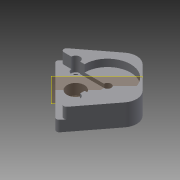
# Autodesk Inventor part: leveling clip
Saved by Autodesk Inventor 2014 (Build 180170000, 170)
## iProperties
Created: 2016-05-11
Part Number: leveling clip
Material: Generic
Document SubType Name: Modeling
Designer: eric.parent
Density: 1 g/cm^3
Appearance: Default
Author: eric.parent
Autodesk Inventor part; units mm, degrees
ref_plane "YZ Plane" through (0, 0, 0) normal (1, 0, 0) x (0, 1, 0)
ref_plane "XZ Plane" through (0, 0, 0) normal (0, 1, 0) x (-1, 0, 0)
ref_plane "XY Plane" through (0, 0, 0) normal (0, 0, 1) x (1, 0, 0)
sketch "Sketch1" plane through (0, 0, 0) normal (0, 0, 1) x (1, 0, 0)
  line L0 (202, 202) -> (202, 0) construction
  line L1 (0, 202) -> (202, 202) construction
  arc A0 (206.2012, 222.0831) -> (193.0425, 222.9456) centre (199.1301, 215.012) ccw projected
  arc A1 (222.9456, 193.0425) -> (222.0831, 206.2012) centre (215.012, 199.1301) ccw projected
  line L2 (206.2012, 222.0831) -> (222.0831, 206.2012)
  line L3 (193.0425, 222.9456) -> (165.7457, 202)
  line L4 (202, 165.7457) -> (222.9456, 193.0425)
  line L5 (165.7457, 202) -> (202, 165.7457)
  point P0 (0, 0)
  constraints: 8 end point, 3 tangent, 2 point on line, 1 parallel
extrude "Extrusion3" add sketch "Sketch1" along normal blind 15
sketch "Sketch3" plane through (0, 0, 15) normal (0, 0, 1) x (1, 0, 0)
  line L0 (165.7457, 202) -> (202, 202)
  line L1 (202, 202) -> (202, 165.7457)
  line L2 (165.7457, 202) -> (202, 165.7457)
  point P0 (0, 0)
  constraints: 6 end point, 1 horizontal, 1 perpendicular
extrude "Extrusion4" cut sketch "Sketch3" against normal blind 7.5
sketch "Sketch5" plane through (0, 0, 15) normal (0, 0, 1) x (1, 0, 0)
  line L0 (222.0831, 206.2012) -> (206.2012, 222.0831) construction
  line L1 (214.1421, 214.1421) -> (134.2284, 134.2284) construction
  line L2 (202, 165.7457) -> (165.7457, 202) construction
  circle A0 centre (190.9439, 190.9439) radius 6
  point P0 (0, 0)
  dimension "d25" = 12
  dimension "d26" = 10
  constraints: 2 end point, 1 centre point, 1 midpoint, 1 perpendicular, 1 point on line
  measures "d25" diameter of A0
  measures "d26" distance from line of L2 A0.centre
extrude "Extrusion6" cut sketch "Sketch5" against normal through all
sketch "Sketch6" plane through (0, 0, 15) normal (0, 0, 1) x (1, 0, 0)
  circle A0 centre (202, 202) radius 2.5
  point P0 (0, 0)
  dimension "d27" = 5
  constraints: 1 centre point, 1 coincident
  measures "d27" diameter of A0
extrude "Extrusion7" cut sketch "Sketch6" against normal through all
sketch "Sketch7" plane through (0, 0, 15) normal (0, 0, 1) x (1, 0, 0)
  arc A0 (202, 199.5) -> (199.5, 202) centre (202, 202) ccw construction
  circle A1 centre (202, 202) radius 16
  point P0 (0, 0)
  dimension "d30" = 32
  constraints: 1 centre point, 1 coincident
  measures "d30" diameter of A1
extrude "Extrusion8" cut sketch "Sketch7" against normal blind 5
sketch "Sketch8" plane through (0, 0, 15) normal (0, 0, 1) x (1, 0, 0)
  line L0 (202, 186) -> (202, 165.7457) construction
  circle A0 centre (190.9439, 190.9439) radius 6 construction
  line L1 (202, 165.7457) -> (165.7457, 202) construction
  line L2 (163.0953, 218.7925) -> (219.2426, 162.6452) construction
  circle A1 centre (202, 179.8878) radius 1.65
  point P0 (0, 0)
  dimension "d33" = 3.3
  constraints: 3 point on line, 2 end point, 1 centre point, 1 parallel
  measures "d33" diameter of A1
extrude "Extrusion9" cut sketch "Sketch8" against normal through all
sketch "Sketch9" plane through (0, 0, 15) normal (0, 0, 1) x (1, 0, 0)
  arc A0 (202, 178.2378) -> (202, 181.5378) centre (202, 179.8878) ccw construction
  circle A1 centre (202, 179.8878) radius 3
  point P0 (0, 0)
  dimension "d36" = 6
  constraints: 1 centre point, 1 coincident
  measures "d36" diameter of A1
extrude "Extrusion10" cut sketch "Sketch9" against normal blind 10
ref_plane "Work Plane1" through (183.8728, 183.8728, 7.5) normal (0.7071068, -0.7071068, 0) x (0, 0, -1)
mirror "Mirror1" about plane through (183.8728, 183.8728, 7.5) normal (0.7071068, -0.7071068, 0) of "Extrusion9", "Extrusion10"
fillet "Fillet6" radius 2 4 edges at (165.7457, 202, 11.25) (165.7457, 202, 3.75) (202, 165.7457, 11.25) (202, 165.7457, 3.75)
body "Solid2"
